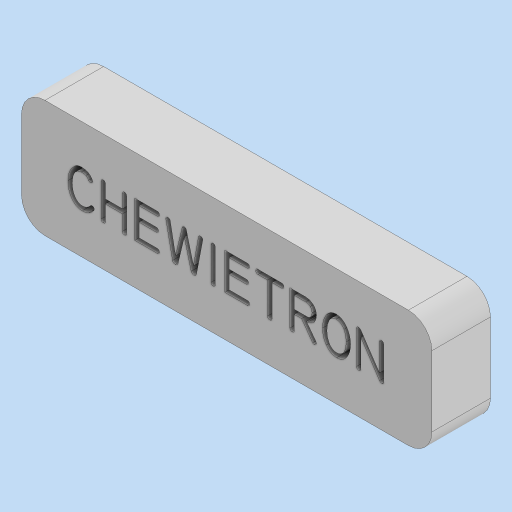
# Autodesk Inventor part: TAG
Saved by Autodesk Inventor 2024 (Build 280153000, 153)
## iProperties
Created: 2024-11-05
Part Number: TAG
Material: Generic
Document SubType Name: Modeling
Designer: MxMon
Density: 1 g/cm^3
Appearance: Default
Author: MxMon
Autodesk Inventor part; units mm, degrees
ref_plane "YZ Plane" through (0, 0, 0) normal (1, 0, 0) x (0, 1, 0)
ref_plane "XZ Plane" through (0, 0, 0) normal (0, 1, 0) x (-1, 0, 0)
ref_plane "XY Plane" through (0, 0, 0) normal (0, 0, 1) x (1, 0, 0)
sketch "Sketch1" plane through (0, 0, 0) normal (0, 0, 1) x (1, 0, 0)
  line L0 (-17.5, 5) -> (17.5, 5)
  line L1 (17.5, 5) -> (17.5, -5)
  line L2 (17.5, -5) -> (-17.5, -5)
  line L3 (-17.5, -5) -> (-17.5, 5)
  line L4 (-17.5, 5) -> (17.5, -5) construction
  line L5 (17.5, 5) -> (-17.5, -5) construction
  point P0 (0, 0)
  dimension "d0" = 35
  dimension "d1" = 10
  constraints: 12 end point, 2 midpoint, 2 parallel, 1 horizontal, 1 perpendicular
  measures "d0" distance of L1.end L2.end
  measures "d1" distance of L0.end L1.end
extrude "Extrusion1" add sketch "Sketch1" along normal blind 5
fillet "Fillet1" radius 2 4 edges at (-17.5, 5, 2.5) (17.5, 5, 2.5) (17.5, -5, 2.5) (-17.5, -5, 2.5)
sketch "Sketch2" plane through (0, 0, 5) normal (0, 0, 1) x (1, 0, 0)
  line L0 (-15.4979, -3.2372) -> (15.4979, -3.2372) construction
  line L1 (15.4979, -3.2372) -> (15.4979, 3.2372) construction
  line L2 (15.4979, 3.2372) -> (-15.4979, 3.2372) construction
  line L3 (-15.4979, 3.2372) -> (-15.4979, -3.2372) construction
  line L4 (15.5, 5) -> (-15.5, 5) projected
  line L5 (17.5, -3) -> (17.5, 3) projected
  spline S0 degree 2 poles (-11.332, -1.0718) (-11.5654, -1.3552) (-11.7797, -1.4576) knots 0 0 0 1 1 1
  spline S1 degree 2 poles (-11.7797, -1.4576) (-12.0108, -1.5743) (-12.3227, -1.5743) knots 0 0 0 1 1 1
  spline S2 degree 2 poles (-12.3227, -1.5743) (-12.8515, -1.5743) (-13.535, -0.6788) (-13.535, 0.0572) knots 0 0 0 1 2 2 2
  spline S3 degree 2 poles (-13.535, 0.0572) (-13.535, 0.8598) (-13.073, 1.298) knots 0 0 0 1 1 1
  spline S4 degree 2 poles (-13.073, 1.298) (-12.8348, 1.6291) (-12.3894, 1.6291) knots 0 0 0 1 1 1
  spline S5 degree 2 poles (-12.3894, 1.6291) (-12.0393, 1.6291) (-11.8155, 1.5124) knots 0 0 0 1 1 1
  spline S6 degree 2 poles (-11.8155, 1.5124) (-11.6202, 1.4171) (-11.4582, 1.1361) knots 0 0 0 1 1 1
  spline S7 degree 2 poles (-11.4582, 1.1361) (-11.4272, 1.086) (-11.4272, 1.0384) knots 0 0 0 1 1 1
  spline S8 degree 2 poles (-11.4272, 1.0384) (-11.4272, 0.967) (-11.5392, 0.8598) (-11.6178, 0.8598) knots 0 0 0 1 2 2 2
  spline S9 degree 2 poles (-11.6178, 0.8598) (-11.7154, 0.8598) (-11.775, 0.9622) knots 0 0 0 1 1 1
  spline S10 degree 2 poles (-11.775, 0.9622) (-11.8726, 1.1289) (-12.0036, 1.1956) knots 0 0 0 1 1 1
  spline S11 degree 2 poles (-12.0036, 1.1956) (-12.1513, 1.2575) (-12.3918, 1.2575) knots 0 0 0 1 1 1
  spline S12 degree 2 poles (-12.3918, 1.2575) (-12.6991, 1.2575) (-12.9086, 0.9979) knots 0 0 0 1 1 1
  spline S13 degree 2 poles (-12.9086, 0.9979) (-13.1706, 0.6764) (-13.1706, 0.0572) knots 0 0 0 1 1 1
  spline S14 degree 2 poles (-13.1706, 0.0572) (-13.1706, -0.5073) (-12.68, -1.2075) (-12.3156, -1.2075) knots 0 0 0 1 2 2 2
  spline S15 degree 2 poles (-12.3156, -1.2075) (-11.9131, -1.2075) (-11.613, -0.8407) knots 0 0 0 1 1 1
  spline S16 degree 2 poles (-11.613, -0.8407) (-11.5582, -0.774) (-11.4796, -0.774) knots 0 0 0 1 1 1
  spline S17 degree 2 poles (-11.4796, -0.774) (-11.4058, -0.774) (-11.2939, -0.886) (-11.2939, -0.9574) knots 0 0 0 1 2 2 2
  spline S18 degree 2 poles (-11.2939, -0.9574) (-11.2939, -1.0217) (-11.332, -1.0718) knots 0 0 0 1 1 1
  spline S19 degree 2 poles (-8.5311, -1.3695) (-8.5311, -1.5576) (-8.7121, -1.5576) knots 0 0 0 1 1 1
  spline S20 degree 2 poles (-8.7121, -1.5576) (-8.8931, -1.5576) (-8.8931, -1.3695) knots 0 0 0 1 1 1
  line L6 (-8.8931, -1.3695) -> (-8.8931, -0.0786)
  line L7 (-8.8931, -0.0786) -> (-10.346, -0.0786)
  line L8 (-10.346, -0.0786) -> (-10.346, -1.3695)
  spline S21 degree 2 poles (-10.346, -1.3695) (-10.346, -1.5576) (-10.527, -1.5576) knots 0 0 0 1 1 1
  spline S22 degree 2 poles (-10.527, -1.5576) (-10.7104, -1.5576) (-10.7104, -1.3695) knots 0 0 0 1 1 1
  line L9 (-10.7104, -1.3695) -> (-10.7104, 1.4147)
  spline S23 degree 2 poles (-10.7104, 1.4147) (-10.7104, 1.6029) (-10.527, 1.6029) knots 0 0 0 1 1 1
  spline S24 degree 2 poles (-10.527, 1.6029) (-10.346, 1.6029) (-10.346, 1.4147) knots 0 0 0 1 1 1
  line L10 (-10.346, 1.4147) -> (-10.346, 0.2929)
  line L11 (-10.346, 0.2929) -> (-8.8931, 0.2929)
  line L12 (-8.8931, 0.2929) -> (-8.8931, 1.4147)
  spline S25 degree 2 poles (-8.8931, 1.4147) (-8.8931, 1.6029) (-8.7121, 1.6029) knots 0 0 0 1 1 1
  spline S26 degree 2 poles (-8.7121, 1.6029) (-8.5311, 1.6029) (-8.5311, 1.4147) knots 0 0 0 1 1 1
  line L13 (-8.5311, 1.4147) -> (-8.5311, -1.3695)
  line L14 (-5.9232, -1.5124) -> (-7.8405, -1.5124)
  line L15 (-7.8405, -1.5124) -> (-7.8405, 1.6029)
  line L16 (-7.8405, 1.6029) -> (-5.9232, 1.6029)
  spline S27 degree 2 poles (-5.9232, 1.6029) (-5.7374, 1.6029) (-5.7374, 1.4195) knots 0 0 0 1 1 1
  spline S28 degree 2 poles (-5.7374, 1.4195) (-5.7374, 1.2313) (-5.9232, 1.2313) knots 0 0 0 1 1 1
  line L17 (-5.9232, 1.2313) -> (-7.4761, 1.2313)
  line L18 (-7.4761, 1.2313) -> (-7.4761, 0.3787)
  line L19 (-7.4761, 0.3787) -> (-6.0161, 0.3787)
  spline S29 degree 2 poles (-6.0161, 0.3787) (-5.8256, 0.3787) (-5.8256, 0.1953) knots 0 0 0 1 1 1
  spline S30 degree 2 poles (-5.8256, 0.1953) (-5.8256, 0.0119) (-6.0161, 0.0119) knots 0 0 0 1 1 1
  line L20 (-6.0161, 0.0119) -> (-7.4761, 0.0119)
  line L21 (-7.4761, 0.0119) -> (-7.4761, -1.1456)
  line L22 (-7.4761, -1.1456) -> (-5.9232, -1.1456)
  spline S31 degree 2 poles (-5.9232, -1.1456) (-5.7374, -1.1456) (-5.7374, -1.329) knots 0 0 0 1 1 1
  spline S32 degree 2 poles (-5.7374, -1.329) (-5.7374, -1.5124) (-5.9232, -1.5124) knots 0 0 0 1 1 1
  line L23 (-2.0387, 1.4195) -> (-2.577, -1.3861)
  spline S33 degree 2 poles (-2.577, -1.3861) (-2.6103, -1.5624) (-2.7913, -1.5624) knots 0 0 0 1 1 1
  spline S34 degree 2 poles (-2.7913, -1.5624) (-2.9795, -1.5624) (-3.0271, -1.3909) knots 0 0 0 1 1 1
  line L24 (-3.0271, -1.3909) -> (-3.613, 0.8622)
  line L25 (-3.613, 0.8622) -> (-4.1536, -1.3885)
  spline S35 degree 2 poles (-4.1536, -1.3885) (-4.1989, -1.5624) (-4.387, -1.5624) knots 0 0 0 1 1 1
  spline S36 degree 2 poles (-4.387, -1.5624) (-4.5799, -1.5624) (-4.6157, -1.3861) knots 0 0 0 1 1 1
  line L26 (-4.6157, -1.3861) -> (-5.1873, 1.4028)
  spline S37 degree 2 poles (-5.1873, 1.4028) (-5.2016, 1.4838) (-5.0849, 1.6029) (-5.0039, 1.6029) knots 0 0 0 1 2 2 2
  spline S38 degree 2 poles (-5.0039, 1.6029) (-4.8467, 1.6029) (-4.8181, 1.4552) knots 0 0 0 1 1 1
  line L27 (-4.8181, 1.4552) -> (-4.3632, -0.9074)
  line L28 (-4.3632, -0.9074) -> (-3.8059, 1.4099)
  spline S39 degree 2 poles (-3.8059, 1.4099) (-3.7702, 1.6029) (-3.6273, 1.6029) knots 0 0 0 1 1 1
  spline S40 degree 2 poles (-3.6273, 1.6029) (-3.4796, 1.6029) (-3.4463, 1.479) knots 0 0 0 1 1 1
  line L29 (-3.4463, 1.479) -> (-2.8342, -0.8907)
  line L30 (-2.8342, -0.8907) -> (-2.4055, 1.4552)
  spline S41 degree 2 poles (-2.4055, 1.4552) (-2.3769, 1.6029) (-2.2292, 1.6029) knots 0 0 0 1 1 1
  spline S42 degree 2 poles (-2.2292, 1.6029) (-2.1411, 1.6029) (-2.0244, 1.4814) (-2.0387, 1.4195) knots 0 0 0 1 2 2 2
  spline S43 degree 2 poles (-0.9741, -1.3647) (-0.9741, -1.5528) (-1.1551, -1.5528) knots 0 0 0 1 1 1
  spline S44 degree 2 poles (-1.1551, -1.5528) (-1.3385, -1.5528) (-1.3385, -1.3647) knots 0 0 0 1 1 1
  line L31 (-1.3385, -1.3647) -> (-1.3385, 1.4195)
  spline S45 degree 2 poles (-1.3385, 1.4195) (-1.3385, 1.6076) (-1.1551, 1.6076) knots 0 0 0 1 1 1
  spline S46 degree 2 poles (-1.1551, 1.6076) (-0.9741, 1.6076) (-0.9741, 1.4195) knots 0 0 0 1 1 1
  line L32 (-0.9741, 1.4195) -> (-0.9741, -1.3647)
  line L33 (1.7601, -1.5124) -> (-0.1572, -1.5124)
  line L34 (-0.1572, -1.5124) -> (-0.1572, 1.6029)
  line L35 (-0.1572, 1.6029) -> (1.7601, 1.6029)
  spline S47 degree 2 poles (1.7601, 1.6029) (1.9458, 1.6029) (1.9458, 1.4195) knots 0 0 0 1 1 1
  spline S48 degree 2 poles (1.9458, 1.4195) (1.9458, 1.2313) (1.7601, 1.2313) knots 0 0 0 1 1 1
  line L36 (1.7601, 1.2313) -> (0.2072, 1.2313)
  line L37 (0.2072, 1.2313) -> (0.2072, 0.3787)
  line L38 (0.2072, 0.3787) -> (1.6672, 0.3787)
  spline S49 degree 2 poles (1.6672, 0.3787) (1.8577, 0.3787) (1.8577, 0.1953) knots 0 0 0 1 1 1
  spline S50 degree 2 poles (1.8577, 0.1953) (1.8577, 0.0119) (1.6672, 0.0119) knots 0 0 0 1 1 1
  line L39 (1.6672, 0.0119) -> (0.2072, 0.0119)
  line L40 (0.2072, 0.0119) -> (0.2072, -1.1456)
  line L41 (0.2072, -1.1456) -> (1.7601, -1.1456)
  spline S51 degree 2 poles (1.7601, -1.1456) (1.9458, -1.1456) (1.9458, -1.329) knots 0 0 0 1 1 1
  spline S52 degree 2 poles (1.9458, -1.329) (1.9458, -1.5124) (1.7601, -1.5124) knots 0 0 0 1 1 1
  line L42 (4.6847, 1.2218) -> (3.8702, 1.2218)
  line L43 (3.8702, 1.2218) -> (3.8702, -1.4409)
  spline S53 degree 2 poles (3.8702, -1.4409) (3.8702, -1.6291) (3.6797, -1.6291) knots 0 0 0 1 1 1
  spline S54 degree 2 poles (3.6797, -1.6291) (3.4915, -1.6291) (3.4915, -1.4409) knots 0 0 0 1 1 1
  line L44 (3.4915, -1.4409) -> (3.4915, 1.2218)
  line L45 (3.4915, 1.2218) -> (2.6746, 1.2218)
  spline S55 degree 2 poles (2.6746, 1.2218) (2.4865, 1.2218) (2.4865, 1.4147) knots 0 0 0 1 1 1
  spline S56 degree 2 poles (2.4865, 1.4147) (2.4865, 1.6029) (2.6746, 1.6029) knots 0 0 0 1 1 1
  line L46 (2.6746, 1.6029) -> (4.6847, 1.6029)
  spline S57 degree 2 poles (4.6847, 1.6029) (4.8753, 1.6029) (4.8753, 1.4147) knots 0 0 0 1 1 1
  spline S58 degree 2 poles (4.8753, 1.4147) (4.8753, 1.2218) (4.6847, 1.2218) knots 0 0 0 1 1 1
  spline S59 degree 2 poles (7.6523, 0.6954) (7.6523, 0.2215) (7.3379, -0.0167) knots 0 0 0 1 1 1
  spline S60 degree 2 poles (7.3379, -0.0167) (7.126, -0.1762) (6.9164, -0.1762) knots 0 0 0 1 1 1
  line L47 (6.9164, -0.1762) -> (6.8068, -0.1762)
  line L48 (6.8068, -0.1762) -> (7.6118, -1.2528)
  spline S61 degree 2 poles (7.6118, -1.2528) (7.6523, -1.3123) (7.6523, -1.3695) knots 0 0 0 1 1 1
  spline S62 degree 2 poles (7.6523, -1.3695) (7.6523, -1.4409) (7.5404, -1.5528) (7.4665, -1.5528) knots 0 0 0 1 2 2 2
  spline S63 degree 2 poles (7.4665, -1.5528) (7.376, -1.5528) (7.3379, -1.4957) knots 0 0 0 1 1 1
  line L49 (7.3379, -1.4957) -> (6.3924, -0.1762)
  line L50 (6.3924, -0.1762) -> (5.766, -0.1762)
  line L51 (5.766, -0.1762) -> (5.766, -1.3647)
  spline S64 degree 2 poles (5.766, -1.3647) (5.766, -1.5528) (5.5802, -1.5528) knots 0 0 0 1 1 1
  spline S65 degree 2 poles (5.5802, -1.5528) (5.3969, -1.5528) (5.3969, -1.3647) knots 0 0 0 1 1 1
  line L52 (5.3969, -1.3647) -> (5.3969, 1.5981)
  line L53 (5.3969, 1.5981) -> (6.7473, 1.5981)
  spline S66 degree 2 poles (6.7473, 1.5981) (7.114, 1.5981) (7.3736, 1.3623) knots 0 0 0 1 1 1
  spline S67 degree 2 poles (7.3736, 1.3623) (7.6523, 1.1075) (7.6523, 0.6954) knots 0 0 0 1 1 1
  spline S68 degree 2 poles (7.2879, 0.6954) (7.2879, 0.9431) (7.126, 1.0932) knots 0 0 0 1 1 1
  spline S69 degree 2 poles (7.126, 1.0932) (6.9711, 1.2313) (6.7473, 1.2313) knots 0 0 0 1 1 1
  line L54 (6.7473, 1.2313) -> (5.766, 1.2313)
  line L55 (5.766, 1.2313) -> (5.766, 0.1953)
  line L56 (5.766, 0.1953) -> (6.9164, 0.1953)
  spline S70 degree 2 poles (6.9164, 0.1953) (7.0164, 0.1953) (7.1283, 0.2906) knots 0 0 0 1 1 1
  spline S71 degree 2 poles (7.1283, 0.2906) (7.2879, 0.4263) (7.2879, 0.6954) knots 0 0 0 1 1 1
  spline S72 degree 2 poles (10.5651, 0.0119) (10.5651, -0.6264) (10.2626, -1.0765) knots 0 0 0 1 1 1
  spline S73 degree 2 poles (10.2626, -1.0765) (9.9268, -1.5743) (9.379, -1.5743) knots 0 0 0 1 1 1
  spline S74 degree 2 poles (9.379, -1.5743) (8.836, -1.5743) (8.493, -1.0765) knots 0 0 0 1 1 1
  spline S75 degree 2 poles (8.493, -1.0765) (8.1763, -0.6192) (8.1763, 0.0119) knots 0 0 0 1 1 1
  spline S76 degree 2 poles (8.1763, 0.0119) (8.1763, 0.6454) (8.474, 1.1122) knots 0 0 0 1 1 1
  spline S77 degree 2 poles (8.474, 1.1122) (8.805, 1.6291) (9.329, 1.6291) knots 0 0 0 1 1 1
  spline S78 degree 2 poles (9.329, 1.6291) (9.8911, 1.6291) (10.2436, 1.1146) knots 0 0 0 1 1 1
  spline S79 degree 2 poles (10.2436, 1.1146) (10.5651, 0.6454) (10.5651, 0.0119) knots 0 0 0 1 1 1
  spline S80 degree 2 poles (10.2007, 0.0119) (10.2007, 0.5144) (10.0078, 0.8455) knots 0 0 0 1 1 1
  spline S81 degree 2 poles (10.0078, 0.8455) (9.7363, 1.2575) (9.329, 1.2575) knots 0 0 0 1 1 1
  spline S82 degree 2 poles (9.329, 1.2575) (8.9551, 1.2575) (8.7407, 0.8693) knots 0 0 0 1 1 1
  spline S83 degree 2 poles (8.7407, 0.8693) (8.5454, 0.524) (8.5454, 0.0119) knots 0 0 0 1 1 1
  spline S84 degree 2 poles (8.5454, 0.0119) (8.5454, -0.4906) (8.7574, -0.836) knots 0 0 0 1 1 1
  spline S85 degree 2 poles (8.7574, -0.836) (8.9884, -1.2075) (9.379, -1.2075) knots 0 0 0 1 1 1
  spline S86 degree 2 poles (9.379, -1.2075) (9.7744, -1.2075) (10.0316, -0.8145) knots 0 0 0 1 1 1
  spline S87 degree 2 poles (10.0316, -0.8145) (10.2007, -0.4954) (10.2007, 0.0119) knots 0 0 0 1 1 1
  spline S88 degree 2 poles (13.3945, -1.379) (13.3945, -1.5576) (13.2397, -1.5576) knots 0 0 0 1 1 1
  spline S89 degree 2 poles (13.2397, -1.5576) (13.1301, -1.5576) (13.0444, -1.4361) knots 0 0 0 1 1 1
  line L57 (13.0444, -1.4361) -> (11.4511, 0.967)
  line L58 (11.4511, 0.967) -> (11.4511, -1.3695)
  spline S90 degree 2 poles (11.4511, -1.3695) (11.4511, -1.5576) (11.2653, -1.5576) knots 0 0 0 1 1 1
  spline S91 degree 2 poles (11.2653, -1.5576) (11.0819, -1.5576) (11.0819, -1.3695) knots 0 0 0 1 1 1
  line L59 (11.0819, -1.3695) -> (11.0819, 1.4385)
  spline S92 degree 2 poles (11.0819, 1.4385) (11.0819, 1.6124) (11.2486, 1.6124) knots 0 0 0 1 1 1
  spline S93 degree 2 poles (11.2486, 1.6124) (11.3677, 1.6124) (11.4511, 1.4909) knots 0 0 0 1 1 1
  line L60 (11.4511, 1.4909) -> (13.0301, -0.8717)
  line L61 (13.0301, -0.8717) -> (13.0301, 1.4242)
  spline S94 degree 2 poles (13.0301, 1.4242) (13.0301, 1.6124) (13.2135, 1.6124) knots 0 0 0 1 1 1
  spline S95 degree 2 poles (13.2135, 1.6124) (13.3945, 1.6124) (13.3945, 1.4242) knots 0 0 0 1 1 1
  line L62 (13.3945, 1.4242) -> (13.3945, -1.379)
  point P0 (0, 0)
  point P1 (0, -3.2372)
  point P2 (0, 5)
  point P3 (15.4979, 0)
  point P4 (17.5, 0)
  constraints: 4 midpoint, 1 horizontal alignment, 1 vertical alignment, 2 other
extrude "Extrusion2" cut sketch "Sketch2" against normal blind 2.5
body "Solid1"
